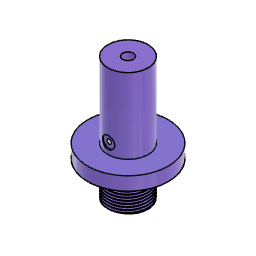
Braço robótico 3.0(cerra 1) v5 (Autodesk Fusion 360 design; units mm, degrees)
Autodesk Fusion 360 part; units mm, degrees
sketch "Sketch4" plane through (0, 0, 0) normal (0, 0, 1) x (1, 0, 0)
  line L0 (-200, 100) -> (-175, 100)
  line L1 (-175, 100) -> (-175, -150)
  line L2 (-175, -150) -> (-200, -150)
  line L3 (-200, -150) -> (-200, 100)
  dimension "d3" = 25
  dimension "d4" = 250
  constraint horizontal L0
  constraint vertical L1
  constraint horizontal L2
  constraint vertical L3
  measures "d3" distance of L0.start L0.end
  measures "d4" distance of L0.start L2.end
sketch "Sketch6" plane through (0, 0, 0) normal (0, 0, 1) x (1, 0, 0)
  circle A0 centre (-151, -158) radius 7.5005
  dimension "d13" = 15.001
  measures "d13" diameter of A0
extrude "Extrude3" add sketch "Sketch6" along normal blind 25 and the other way blind 8 makes body 1
sketch "Sketch7" plane through (0, 0, 25) normal (0, 0, 1) x (-1, 0, 0)
  circle A0 centre (151, 158) radius 7.5005
  circle A1 centre (151, 158) radius 7.5005
  constraint concentric A0 A1
extrude "Extrude4" add sketch "Sketch7" along normal blind 13 separate body makes body 2
thread "Thread1" "ISO Metric profile 15.0 M15x1 6g" major diameter 14.884 minor diameter 13.7405 pitch 1 angle 60 modelled right hand crest width 0.1426 on face at (-155.0694, -164.3006, 33.6667) crest through (-158.442, -158, 24.75) on bodies 2
sketch "Sketch8" plane through (0, 0, 25) normal (0, 0, 1) x (-1, 0, 0)
  circle A0 centre (151, 158) radius 7.5005
  circle A1 centre (151, 158) radius 15
  dimension "d18" = 30
  constraint concentric A0 A1
  measures "d18" diameter of A1
extrude "Extrude5" add sketch "Sketch8" against normal blind 5 bodies 1
move_body "Move1" bodies 1 2 to x (1, 0, 0) y (0, -1, 0) z (0, 0, -1) at (0, -346, -16)
move_body "Move2" bodies 2 1 to x (1, 0, 0) y (0, 1, 0) z (0, 0, 1) at (15.7718, 32.1984, 41.8608)
sketch "Sketch9" plane through (0, 0, 33.8608) normal (0, 0, 1) x (-1, 0, 0)
  circle A0 centre (135.2282, 155.8016) radius 7.5005
  circle A1 centre (135.2282, 155.8016) radius 2.0005
  dimension "d23" = 4.001
  constraint concentric A0 A1
  measures "d23" diameter of A1
extrude "Extrude6" cut sketch "Sketch9" against normal blind 10 contours A1 bodies 1
move_body "Move3" bodies 1 2 to x (1, 0, 0) y (0, 1, 0) z (0, 0, 1) at (122.2616, -14.6951, 14.3874)
extrude "Extrude7" cut 1 faces at (-12.4512, -169.9753, 38.2482) along direction (0, 0, -1) blind 18 on bodies 1 bodies 1
sketch "Sketch12" plane through (0, 0, 20.2482) normal (0, 0, 1) x (-1, 0, 0)
  circle A0 centre (12.9666, 170.4967) radius 7.5005
  circle A1 centre (12.9666, 170.4967) radius 15
hole "Hole1" at (-12.9666, -177.9972, 24.1805) direction (0, 1, 0) diameter 1.623 depth 50 tip angle 180 counterbore diameter 4.5 counterbore depth 0.5 bodies 1
thread "Thread2" "ISO Metric profile 2.0 M2x0.4 6H"
component "4124A15_7-1 4 Diameter Smooth-Cut Circular Saw Blade for Wood" placed x (1, 0, 0) y (0, 1, 0) z (0, 0, 1) at (0, 0, 0)
component "6343K96_Bearing Locknut" placed x (1, 0, 0) y (0, 0, -1) z (0, 1, 0) at (-164.7507, -187.0518, -22.2618)
component "6627T34_Stepper Motor" placed x (1, 0, 0) y (0, 1, 0) z (0, 0, 1) at (-161.9415, -183.813, -21.8716)
